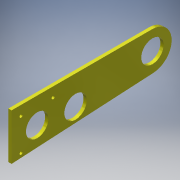
# Autodesk Inventor part: Hopper pully plate
Saved by Autodesk Inventor 2017 (Build 210142000, 142)
## iProperties
Created: 2017-01-14
Part Number: Hopper pully plate
Material: Generic
Document SubType Name: Modeling
Designer: Ben
Density: 1 g/cm^3
Appearance: Smooth - Yellow
Author: Ben
Autodesk Inventor part; units mm, degrees
ref_plane "YZ Plane" through (0, 0, 0) normal (1, 0, 0) x (0, 1, 0)
ref_plane "XZ Plane" through (0, 0, 0) normal (0, 1, 0) x (-1, 0, 0)
ref_plane "XY Plane" through (0, 0, 0) normal (0, 0, 1) x (1, 0, 0)
sketch "Sketch1" plane through (0, 0, 0) normal (1, 0, 0) x (0, 1, 0)
  line L0 (25.4, 25.4) -> (25.4, -114.1235)
  arc A0 (-12.6706, -115.1818) -> (25.4, -114.1235) centre (6.35, -114.1235) ccw
  line L1 (-20.4928, 25.4) -> (-12.6706, -115.1818)
  circle A1 centre (0, 0) radius 11.1125
  circle A2 centre (6.35, -114.1235) radius 11.1125
  line L2 (6.35, -114.1235) -> (0, 0) construction
  line L3 (25.4, 25.4) -> (-20.4928, 25.4)
  circle A3 centre (-3.175, -37.9675) radius 11.1125
  circle A4 centre (6.35, -114.1235) radius 9.525 construction
  circle A5 centre (6.35, -114.1235) radius 15.875 construction
  line L4 (15.875, -15.875) -> (15.875, 15.875) construction
  line L5 (15.875, 15.875) -> (-15.875, 15.875) construction
  circle A6 centre (15.875, 15.875) radius 1.5875
  circle A7 centre (-15.875, 15.875) radius 1.5875
  circle A8 centre (15.875, -15.875) radius 1.5875
  point P0 (6.8794, -133.1661)
  dimension "d1" = 114.3
  dimension "d2" = 6.35
  dimension "d3" = 22.225
  dimension "d9" = 25.4
  dimension "d10" = 25.4
  dimension "d11" = 19.05
  dimension "d12" = 38.1
  dimension "d13" = 3.175
  dimension "d14" = 19.05
  dimension "d15" = 6.35
  dimension "d25" = 3.175
  dimension "d26" = 9.525
  dimension "d27" = 9.525
  dimension "d28" = 31.75
  constraints: 13 end point, 9 centre point, 7 coincident, 4 equal radius, 3 point on circle, 2 perpendicular, 2 tangent, 2 vertical, 1 horizontal
  measures "d1" distance of point (0, 0) A0.centre
  measures "d2" horizontal distance of A0.centre point (0, 0)
  measures "d3" diameter of A1
  measures "d9" distance from line of L0 point (0, 0)
  measures "d10" distance from line of point (0, 0) L3
  measures "d11" distance from line of point (0, 0) L1
  measures "d12" distance of point (0, 0) A3.centre
  measures "d13" horizontal distance of point (0, 0) A3.centre
  measures "d14" diameter of A4
  measures "d15" radial gap between concentric circles of A5 A4
  measures "d25" diameter of A6
  measures "d26" distance between parallel lines of L0 L4
  measures "d27" distance between parallel lines of L3 L5
  measures "d28" distance of L4.start L4.end
extrude "Extrusion1" add sketch "Sketch1" along normal blind 3.175
body "Solid1"
